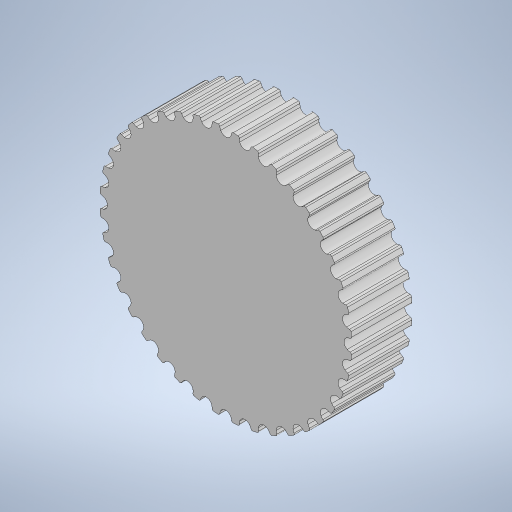
# Autodesk Inventor part: GT2 Belt Generator
Saved by Autodesk Inventor 2023.4 (Build 274418000, 418)
## iProperties
Created: 2024-06-27
Part Number: GT2 Belt Generator
Material: Generic
Document SubType Name: Modeling
Designer: Nathan Cai
Density: 1 g/cm^3
Appearance: Default
Author: Nathan Cai
Autodesk Inventor part; units mm, degrees
ref_plane "YZ Plane" through (0, 0, 0) normal (1, 0, 0) x (0, 1, 0)
ref_plane "XZ Plane" through (0, 0, 0) normal (0, 1, 0) x (-1, 0, 0)
ref_plane "XY Plane" through (0, 0, 0) normal (0, 0, 1) x (1, 0, 0)
sketch "Sketch1" plane through (0, 0, 0) normal (0, 0, 1) x (1, 0, 0)
  circle A0 centre (0, 0) radius 12.7324 construction
  circle A1 centre (0, 0) radius 12.4784
  circle A2 centre (0, 0) radius 13.1084
  line L0 (0, 0) -> (0, 13.1084) construction
  arc A3 (0, 11.7284) -> (0.4989, 12.0402) centre (0, 12.2834) ccw
  line L1 (0, 12.4784) -> (-0.6715, 12.4784) construction
  arc A4 (0.4989, 12.0402) -> (0.5887, 12.3288) centre (-0.4, 12.4784) ccw
  arc A5 (0.746, 12.4561) -> (0.5887, 12.3288) centre (0.7371, 12.3063) ccw
  arc A6 (-0.4989, 12.0402) -> (0, 11.7284) centre (0, 12.2834) ccw
  arc A7 (-0.5887, 12.3288) -> (-0.4989, 12.0402) centre (0.4, 12.4784) ccw
  arc A8 (-0.5887, 12.3288) -> (-0.746, 12.4561) centre (-0.7371, 12.3063) ccw
  point P0 (-0.746, 12.4561)
  dimension "d0" = 25.4648
  dimension "PLD" = 0.254
  dimension "i" = 0.63
  dimension "R3" = 0.555
  dimension "th" = 0.75
  dimension "tb" = 0.4
  dimension "R2" = 1
  dimension "R1" = 0.15
  constraints: 14 point on circle, 8 centre point, 5 symmetric about line, 4 end point, 3 coincident, 3 point on line, 3 tangent, 1 line through centre, 1 perpendicular, 1 vertical, 1 vertical alignment, 5 other
  measures "d0" diameter of A0
  measures "PLD" radial gap between concentric circles of A0 A1
  measures "R3" radius of A3
  measures "th" distance from line of A3.start L1
  measures "tb" distance from line of L0 A4.centre
  measures "R2" radius of A4
  measures "R1" radius of A5
extrude "Extrusion1" add sketch "Sketch1" along normal blind 6 contours A1 A8 A7 A6 A3 A4 A5 | A5 A4 A3 A6 A7 A8 A1
extrude "Extrusion2" cut sketch "Sketch1" along normal through all contours A5 A4 A3 A6 A7 A8 A1 picked at (0, 12.2267)
pattern_circular "Circular Pattern1" count 40 over 360 about axis through (0, 0, 0) along (0, 0, 1) of "Extrusion2"
equation "\"d3\" = width"
equation "\"pitch\" = 2"
equation "\"width\" = 6"
body "Solid1"
